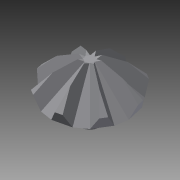
# Autodesk Inventor part: Beveled_Gear
Saved by Autodesk Inventor 2015 (Build 190159000, 159)
## iProperties
Created: 2016-02-12
Part Number: Beveled_Gear
Material: Generic
Document SubType Name: Modeling
Designer: david_000
Density: 1 g/cm^3
Appearance: Default
Author: david_000
Autodesk Inventor part; units mm, degrees
ref_plane "YZ Plane" through (0, 0, 0) normal (1, 0, 0) x (0, 1, 0)
ref_plane "XZ Plane" through (0, 0, 0) normal (0, 1, 0) x (-1, 0, 0)
ref_plane "XY Plane" through (0, 0, 0) normal (0, 0, 1) x (1, 0, 0)
sketch "Sketch7" plane through (0, 0, 0) normal (0, 1, 0) x (-1, 0, 0)
  line L0 (0, 0) -> (-22.225, 0)
  line L1 (0, 0) -> (-15.7154, -15.7154) construction
  line L2 (0, 0) -> (-22.225, 0) construction
  line L3 (-22.225, 0) -> (-19.8975, -9.9016)
  line L4 (-19.8975, -9.9016) -> (-15.7154, -15.7154)
  line L5 (-15.7154, -15.7154) -> (0, 0)
  dimension "d25" = 22.225
  dimension "d26" = 45
  constraints: 12 end point, 1 coincident, 1 collinear, 1 horizontal
  measures "d25" distance of L0.start L0.end
  measures "d26" angle of L2 L1
extrude "Extrusion6" add sketch "Sketch7" along normal blind 19.05
chamfer "Chamfer2" distance 19.05 angle 45 2 edges at (17.8065, 19.05, -12.8085) (21.0612, 19.05, -4.9508)
pattern_circular "Circular Pattern3" count 8 over 360 about axis through (0, 0, 0) along (0, 1, 0) of "Extrusion6", "Chamfer2"
sketch "Sketch8" plane through (-15.7154, 0, -15.7154) normal (-0.6011477, 0.7071068, -0.372319) x (0.5066767, 0.6975367, 0.5066767)
  line L0 (0, 0) -> (1.6678, -10.0338)
  line L1 (1.6678, -10.0338) -> (27.6226, -1.8784)
  line L2 (27.6226, -1.8784) -> (1.6678, -10.0338) projected
  line L3 (27.6226, -1.8784) -> (27.3104, 0)
  line L4 (27.3104, 0) -> (0, 0)
  line L5 (0, 0) -> (27.3104, 0) projected
  point P0 (15.9253, -2.5084)
  constraints: 8 end point, 2 collinear
extrude "Extrusion7" add sketch "Sketch8" along normal blind 6.35 draft -23.6
sketch "Sketch9" plane through (0, 0, 0) normal (0, -1, 0) x (1, 0, 0)
  circle A0 centre (0, 0) radius 4.7625
  dimension "d37" = 9.525
  constraints: 1 centre point, 1 coincident
  measures "d37" diameter of A0
extrude "Extrusion8" add sketch "Sketch9" along normal blind 12.7
pattern_circular "Circular Pattern4" count 8 over 360 about axis through (0, 0, 0) along (0, -1, 0) of "Extrusion7"
body "Solid4"
